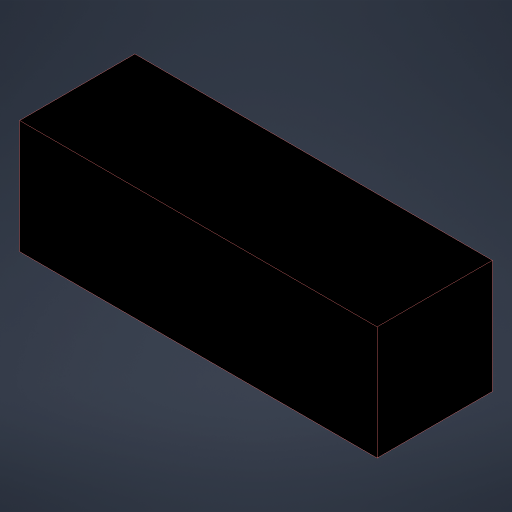
# Autodesk Inventor part: battery
Saved by Autodesk Inventor 2023.2 (Build 272271000, 271)
## iProperties
Created: 2023-01-07
Part Number: battery
Material: Battery
Document SubType Name: Modeling
Designer: Maciej
Density: 2.03 g/cm^3
Appearance: Generic
Author: Maciej
Autodesk Inventor part; units mm, degrees
ref_plane "YZ Plane" through (0, 0, 0) normal (1, 0, 0) x (0, 1, 0)
ref_plane "XZ Plane" through (0, 0, 0) normal (0, 1, 0) x (-1, 0, 0)
ref_plane "XY Plane" through (0, 0, 0) normal (0, 0, 1) x (1, 0, 0)
sketch "Sketch1" plane through (0, 0, 0) normal (0, 1, 0) x (-1, 0, 0)
  line L0 (0, 0) -> (-107, 0)
  line L1 (-107, 0) -> (-107, -34.5)
  line L2 (-107, -34.5) -> (0, -34.5)
  line L3 (0, -34.5) -> (0, 0)
  dimension "d0" = 107
  dimension "d1" = 34.5
  constraints: 8 end point, 2 parallel, 1 horizontal, 1 perpendicular
  measures "d0" distance of L2.end L1.end
  measures "d1" distance of L1.end L0.end
extrude "Extrusion1" add sketch "Sketch1" along normal blind 34
body "Solid1"
